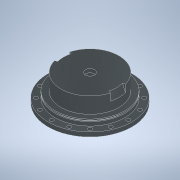
# Autodesk Inventor part: Крышка цилиндра 2
Saved by Autodesk Inventor 2021 (Build 250183000, 183)
## iProperties
Created: 2020-11-05
Part Number: Крышка цилиндра 2
Material: Чугун, литейный
Document SubType Name: Modeling
Designer: Тимоха
Density: 7.15 g/cm^3
Appearance: Чугун серый
Mass: 217332 g
Surface Area: 10065.2 cm^2
Volume: 30396 cm^3
Author: Тимоха
Autodesk Inventor part; units mm, degrees
ref_plane "YZ Plane" through (0, 0, 0) normal (1, 0, 0) x (0, 1, 0)
ref_plane "XZ Plane" through (0, 0, 0) normal (0, 1, 0) x (-1, 0, 0)
ref_plane "XY Plane" through (0, 0, 0) normal (0, 0, 1) x (1, 0, 0)
sketch "Эскиз1" plane through (0, 0, 0) normal (0, 0, 1) x (1, 0, 0)
  line L0 (70, 0) -> (70, 160)
  line L1 (70, 160) -> (32, 160)
  line L2 (32, 160) -> (32, 185)
  line L3 (32, 185) -> (200, 185)
  line L4 (200, 185) -> (200, 75)
  line L5 (200, 75) -> (240, 75)
  line L6 (240, 75) -> (240, 33)
  line L7 (240, 33) -> (290, 33)
  line L8 (240, 67.4515) -> (232, 67.4515)
  line L9 (232, 67.4515) -> (232, 59.4515)
  line L10 (232, 59.4515) -> (240, 59.4515)
  line L11 (290, 33) -> (290, 3)
  line L12 (105, 0) -> (105, 0)
  line L13 (105, 0) -> (70, 0)
  line L14 (0, -68.2) -> (0, 227.2) projected
  line L15 (70, 0) -> (105, 0)
  line L16 (105, 0) -> (105, -26)
  line L17 (105, -26) -> (240, -26)
  line L18 (240, -26) -> (240, 3)
  line L19 (240, 3) -> (290, 3)
  line L20 (32, 160) -> (49, 160)
  line L21 (49, 160) -> (49, 159)
  circle A0 centre (49, 159) radius 3
  point P0 (0, 0)
  point P1 (46.1716, 160)
  point P2 (51.8284, 160)
  dimension "d0" = 70
  dimension "d1" = 160
  dimension "d2" = 38
  dimension "d3" = 25
  dimension "d4" = 168
  dimension "d5" = 110
  dimension "d6" = 40
  dimension "d7" = 42
  dimension "d8" = 50
  dimension "d9" = 8
  dimension "d10" = 8
  dimension "d11" = 30
  dimension "d14" = 105
  dimension "d15" = 26
  dimension "d109" = 1
  constraints: 42 end point, 10 perpendicular, 4 vertical, 3 horizontal, 3 point on line, 1 centre point, 1 coincident, 1 collinear
  measures "d0" distance of L0.start point (0, 0)
  measures "d1" distance of L0.start L0.end
  measures "d2" distance of L0.end L1.end
  measures "d3" distance of L1.end L2.end
  measures "d4" distance of L2.end L3.end
  measures "d5" distance of L3.end L4.end
  measures "d6" distance of L4.end L5.end
  measures "d7" distance of L5.end L6.end
  measures "d8" distance of L6.end L7.end
  measures "d9" distance of L8.start L8.end
  measures "d10" distance of L8.end L9.end
  measures "d11" distance of L7.end L11.end
  measures "d14" distance of point (0, 0) L12.end
  measures "d15" distance of L12.end L16.end
  measures "d109" distance of L20.end L21.end
revolve "Вращение1" add sketch "Эскиз1" angle 360 about axis through (0, -10, 0) along (0, 1, 0) contours L0 L1 A0 L2 L3 L4 L5 L6 L8 L9 L10 L7 L11 L19 L18 L17 L16 L13
sketch "Эскиз2" plane through (0, 0, 0) normal (0, 0, 1) x (1, 0, 0)
  line L0 (-200, 185) -> (-200, 75) projected
  line L1 (-200, 185) -> (200, 185) projected
  line L2 (-200, 185) -> (-200, 146)
  line L3 (0, -37) -> (0, 222) projected
  line L4 (-206, 115) -> (-200, 135)
  line L5 (-200, 135) -> (-183.4896, 185)
  point P0 (0, 0)
  constraints: 6 end point, 2 point on line, 3 other
revolve "Вращение2" cut sketch "Эскиз2" angle 30 mid plane about axis through (0, -10, 0) along (0, 1, 0)
pattern_circular "Круговой массив1" count 2 over 360 about axis through (0, -10, 0) along (0, 1, 0) of "Вращение2"
sketch "Эскиз3" plane through (0, 3, 0) normal (0, -1, 0) x (1, 0, 0)
  circle A0 centre (0, 0) radius 290 projected
  line L0 (-290, 0) -> (-265, 0)
  dimension "d21" = 25
  constraints: 2 end point, 1 horizontal, 1 horizontal alignment, 1 other
  measures "d21" distance of L0.start L0.end
hole "Отверстие1" at (-265, 3, 0) direction (0, 1, 0) diameter 26 end through all
pattern_circular "Круговой массив2" count 16 over 360 about axis through (0, -10, 0) along (0, 1, 0) of "Отверстие1"
sketch "Эскиз4" plane through (0, 0, 0) normal (0, -1, 0) x (1, 0, 0)
  circle A0 centre (0, 0) radius 70 projected
  line L0 (0, -70) -> (0, -87.5)
  dimension "d32" = 17.5
  constraints: 2 end point, 1 vertical, 1 vertical alignment, 1 other
  measures "d32" distance of L0.start L0.end
hole "Отверстие2" at (0, 0, -87.5) direction (0, 1, 0) diameter 8 depth 20 tip angle 118 counterbore diameter 10 counterbore depth 15
pattern_circular "Круговой массив3" count 10 over 360 about axis through (0, 80, 0) along (0, -1, 0) of "Отверстие2"
thread "Резьба1" size "M10x1.5" class "6H" standard "ANSI Metric M Profile" full length
thread "Резьба2" size "M10x1.5" class "6H" standard "ANSI Metric M Profile" full length
thread "Резьба3" size "M10x1.5" class "6H" standard "ANSI Metric M Profile" full length
thread "Резьба4" size "M10x1.5" class "6H" standard "ANSI Metric M Profile" full length
thread "Резьба5" size "M10x1.5" class "6H" standard "ANSI Metric M Profile" full length
thread "Резьба6" size "M10x1.5" class "6H" standard "ANSI Metric M Profile" full length
thread "Резьба7" size "M10x1.5" class "6H" standard "ANSI Metric M Profile" full length
thread "Резьба8" size "M10x1.5" class "6H" standard "ANSI Metric M Profile" full length
thread "Резьба9" size "M10x1.5" class "6H" standard "ANSI Metric M Profile" full length
thread "Резьба10" size "M10x1.5" class "6H" standard "ANSI Metric M Profile" full length
sketch "Эскиз5" plane through (0, -26, 0) normal (0, -1, 0) x (1, 0, 0)
  line L0 (0, 0) -> (-205, 0)
  dimension "d63" = 205
  constraints: 2 end point, 1 horizontal
  measures "d63" distance of L0.start L0.end
hole "Отверстие3" at (-205, -26, 0) direction (0, 1, 0) diameter 18 depth 60 tip angle 118 counterbore diameter 20 counterbore depth 50
pattern_circular "Круговой массив4" count 16 over 360 about axis through (0, -13, 0) along (0, -1, 0) of "Отверстие3"
thread "Резьба11" size "M20x2.5" class "6H" standard "ANSI Metric M Profile" full length
thread "Резьба12" size "M20x2.5" class "6H" standard "ANSI Metric M Profile" full length
thread "Резьба13" size "M20x2.5" class "6H" standard "ANSI Metric M Profile" full length
thread "Резьба14" size "M20x2.5" class "6H" standard "ANSI Metric M Profile" full length
thread "Резьба15" size "M20x2.5" class "6H" standard "ANSI Metric M Profile" full length
thread "Резьба16" size "M20x2.5" class "6H" standard "ANSI Metric M Profile" full length
thread "Резьба17" size "M20x2.5" class "6H" standard "ANSI Metric M Profile" full length
thread "Резьба18" size "M20x2.5" class "6H" standard "ANSI Metric M Profile" full length
thread "Резьба19" size "M20x2.5" class "6H" standard "ANSI Metric M Profile" full length
thread "Резьба20" size "M20x2.5" class "6H" standard "ANSI Metric M Profile" full length
thread "Резьба21" size "M20x2.5" class "6H" standard "ANSI Metric M Profile" full length
thread "Резьба22" size "M20x2.5" class "6H" standard "ANSI Metric M Profile" full length
thread "Резьба23" size "M20x2.5" class "6H" standard "ANSI Metric M Profile" full length
thread "Резьба24" size "M20x2.5" class "6H" standard "ANSI Metric M Profile" full length
thread "Резьба25" size "M20x2.5" class "6H" standard "ANSI Metric M Profile" full length
thread "Резьба26" size "M20x2.5" class "6H" standard "ANSI Metric M Profile" full length
sketch "Эскиз6" plane through (0, -26, 0) normal (0, -1, 0) x (1, 0, 0)
  circle A0 centre (0, 0) radius 240 projected
  circle A1 centre (0, 0) radius 230
  dimension "d106" = 460
  constraints: 1 centre point, 1 coincident
  measures "d106" diameter of A1
extrude "Выдавливание1" cut sketch "Эскиз6" against normal blind 10
